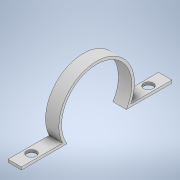
# Autodesk Inventor part: part7
Saved by Autodesk Inventor 2021 (Build 250183000, 183)
## iProperties
Created: 2022-12-10
Part Number: part7
Material: Generic
Document SubType Name: Modeling
Designer: user
Density: 1 g/cm^3
Appearance: Default
Author: user
Autodesk Inventor part; units mm, degrees
ref_plane "YZ Plane" through (0, 0, 0) normal (1, 0, 0) x (0, 1, 0)
ref_plane "XZ Plane" through (0, 0, 0) normal (0, 1, 0) x (-1, 0, 0)
ref_plane "XY Plane" through (0, 0, 0) normal (0, 0, 1) x (1, 0, 0)
sketch "Sketch9" plane through (0, 0, 0) normal (1, 0, 0) x (0, 1, 0)
  arc A0 (-11.2991, -17.7011) -> (-11.2991, 17.7011) centre (0, 0) ccw
  arc A1 (-9.6991, -20.4129) -> (-9.6991, 20.4129) centre (0, 0) ccw
  line L0 (-9.6991, 45) -> (-11.2991, 45)
  line L1 (-11.2991, 45) -> (-11.2991, 17.7011)
  line L2 (-9.6991, 0) -> (-16.1126, 0) construction
  line L3 (-9.6991, -45) -> (-11.2991, -45)
  line L4 (-11.2991, -45) -> (-11.2991, -17.7011)
  line L5 (-9.6991, 45) -> (-9.6991, 18.626)
  line L6 (-9.6991, -18.626) -> (-9.6991, -45)
  dimension "d36" = 42
  dimension "d37" = 45.2
  dimension "d38" = 90
  dimension "d39" = 45
  dimension "d40" = 1.6
  constraints: 14 end point, 6 point on circle, 3 point on line, 2 centre point, 2 coincident, 2 horizontal, 2 symmetric about line, 2 vertical, 1 perpendicular
  measures "d36" diameter of A0
  measures "d37" diameter of A1
  measures "d38" distance of L0.start L3.start
  measures "d39" vertical distance of point (0, 0) L3.start
  measures "d40" distance of L0.start L0.end
extrude "Extrusion5" add sketch "Sketch9" along normal blind 8
sketch "Sketch10" plane through (0, -9.6991, 45) normal (0, 1, 0) x (1, 0, 0)
  circle A0 centre (4, 10) radius 2.9
  circle A1 centre (4, 80) radius 2.9
  line L0 (0, 0) -> (8, 0) projected
  line L1 (0, 90) -> (8, 90) projected
  line L2 (8, 90) -> (8, 65.4129) projected
  line L3 (0, 24.5871) -> (0, 0) projected
  point P0 (0, 45)
  dimension "d43" = 5.8
  dimension "d44" = 5.8
  dimension "d45" = 10
  dimension "d46" = 10
  dimension "d47" = 4
  dimension "d48" = 4
  constraints: 2 centre point
  measures "d43" diameter of A0
  measures "d44" diameter of A1
  measures "d45" distance from line of A0.centre L0
  measures "d46" distance from line of L1 A1.centre
  measures "d47" distance from line of L2 A1.centre
  measures "d48" distance from line of L3 A0.centre
extrude "Extrusion6" cut sketch "Sketch10" against normal through all
body "Solid4"
